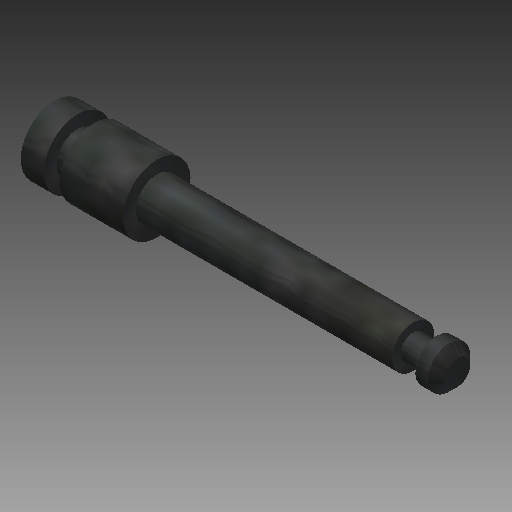
# Autodesk Inventor part: 403-13
Saved by Autodesk Inventor 2019 (Build 230136000, 136)
## iProperties
Company: Autodesk Inc.
Created: 2017-06-27
Part Number: 403-13
Material: Steel
Document SubType Name: Modeling
Designer: Autodesk Inc.
Mass: 0.607988 g
Surface Area: 1.60928 cm^2
Volume: 0.0774507 cm^3
Density: 7.85 g/cm^3
Appearance: Plate
Author: Inventor
Autodesk Inventor part; units mm, degrees
ref_plane "YZ Plane" through (0, 0, 0) normal (1, 0, 0) x (0, 1, 0)
ref_plane "XZ Plane" through (0, 0, 0) normal (0, 1, 0) x (-1, 0, 0)
ref_plane "XY Plane" through (0, 0, 0) normal (0, 0, 1) x (1, 0, 0)
sketch "Sketch1" plane through (0, 0, 0) normal (0, 0, 1) x (1, 0, 0)
  line L0 (0, 0) -> (1.1, 0)
  line L1 (1.1, 0) -> (1.1, 1.6)
  line L2 (1.1, 1.6) -> (0, 1.6)
  line L3 (0, 1.6) -> (0, 0)
  line L4 (1.1, 0) -> (1.85, 0)
  line L5 (1.85, 0) -> (1.85, 1)
  line L6 (1.85, 1) -> (1.1, 1)
  line L7 (1.1, 1) -> (1.1, 0)
  line L8 (1.85, 0) -> (4.85, 0)
  line L9 (4.85, 0) -> (4.85, 1.6)
  line L10 (4.85, 1.6) -> (1.85, 1.6)
  line L11 (1.85, 1.6) -> (1.85, 0)
  line L12 (4.85, 0) -> (17, 0)
  line L13 (17, 0) -> (17, 1)
  line L14 (17, 1) -> (4.85, 1)
  line L15 (4.85, 1) -> (4.85, 0)
  line L16 (17, 0) -> (18.1, 0)
  line L17 (18.1, 0) -> (18.1, 0.6)
  line L18 (18.1, 0.6) -> (17, 0.6)
  line L19 (17, 0.6) -> (17, 0)
  line L20 (18.1, 0) -> (19.1, 0)
  line L21 (19.1, 0) -> (19.1, 1)
  line L22 (19.1, 1) -> (18.1, 1)
  line L23 (18.1, 1) -> (18.1, 0)
  dimension "d0" = 1.1
  dimension "d1" = 1.85
  dimension "d2" = 4.85
  dimension "d3" = 19.1
  dimension "d4" = 18.1
  dimension "d5" = 17
  dimension "d6" = 2
  dimension "d7" = 1.2
  dimension "d8" = 3.2
  dimension "d9" = 2
  constraints: 48 end point, 12 parallel, 6 horizontal, 6 perpendicular, 2 collinear
  measures "d0" distance of L1.end L2.end
  measures "d1" distance between parallel lines of L11 L3
  measures "d2" distance between parallel lines of L9 L3
  measures "d3" distance between parallel lines of L21 L3
  measures "d4" distance between parallel lines of L23 L3
  measures "d5" distance between parallel lines of L13 L3
  measures "d6" diameter of L22 L20
  measures "d7" diameter of L18 L20
  measures "d8" diameter of L2 L0
  measures "d9" diameter of L6 L0
revolve "Revolution1" add sketch "Sketch1" angle 360 about axis through (0, 0, 0) along (1, 0, 0)
chamfer "Chamfer1" distance 0.4 angle 45 1 edges at (19.1, -1, 0)
body "Solid1"
